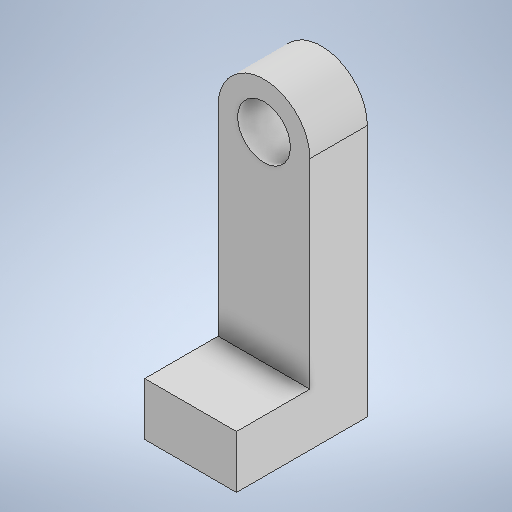
# Autodesk Inventor part: Podstawa
Saved by Autodesk Inventor 2025 (Build 290162000, 162)
## iProperties
Created: 2025-05-28
Part Number: Podstawa
Material: Ogólny
Document SubType Name: Modeling
Designer: tjaku
Density: 1 g/cm^3
Appearance: Domyślna
Author: tjaku
Autodesk Inventor part; units mm, degrees
ref_plane "YZ Plane" through (0, 0, 0) normal (1, 0, 0) x (0, 1, 0)
ref_plane "XZ Plane" through (0, 0, 0) normal (0, 1, 0) x (-1, 0, 0)
ref_plane "XY Plane" through (0, 0, 0) normal (0, 0, 1) x (1, 0, 0)
sketch "Szkic1" plane through (0, 0, 0) normal (0, 0, 1) x (1, 0, 0)
  line L0 (0, 0) -> (40, 0)
  line L1 (40, 0) -> (40, 110)
  line L2 (40, 110) -> (0, 110)
  line L3 (0, 110) -> (0, 0)
  circle A0 centre (20, 110) radius 11.5
  circle A1 centre (20, 110) radius 20
  dimension "d0" = 40
  dimension "d1" = 110
  dimension "d2" = 23
  constraints: 8 end point, 3 perpendicular, 1 centre point, 1 coincident, 1 horizontal, 1 midpoint, 3 other
  measures "d0" distance of L0.start L0.end
  measures "d1" distance of L0.end L1.end
  measures "d2" diameter of A0
extrude "Wyciągnięcie proste1" add sketch "Szkic1" along normal blind 25 contours L3 A1 L1 L0 | A1 L2 A0 | L2 A0 A1
sketch "Szkic2" plane through (0, 0, 25) normal (0, 0, 1) x (1, 0, 0)
  line L0 (0, 110) -> (0, 0) projected
  line L1 (0, 0) -> (0, 23)
  line L2 (0, 23) -> (40, 23)
  line L3 (40, 0) -> (40, 110) projected
  line L4 (40, 23) -> (40, 0)
  line L5 (40, 0) -> (0, 0)
  dimension "d5" = 23
  dimension "d6" = 40
  constraints: 8 end point, 2 point on line, 1 collinear, 1 perpendicular
  measures "d5" distance of L0.end L1.end
  measures "d6" distance of L1.end L2.end
extrude "Wyciągnięcie proste2" add sketch "Szkic2" along normal blind 32
